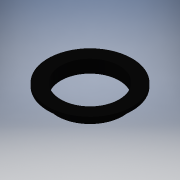
# Autodesk Inventor part: オイレスF　d25-D28-l12
Saved by Autodesk Inventor 2017.3 (Build 213256000, 256)
## iProperties
Created: 2017-03-06
Part Number: オイレスF　d25-D28-l12
Material: アセタール樹脂、黒
Document SubType Name: Modeling
Designer: 大空
Density: 1.425 g/cm^3
Appearance: 滑らか - 黒
Mass: 1.83827 g
Surface Area: 20.0748 cm^2
Volume: 1.29002 cm^3
Author: 大空
Autodesk Inventor part; units mm, degrees
ref_plane "YZ Plane" through (0, 0, 0) normal (1, 0, 0) x (0, 1, 0)
ref_plane "XZ Plane" through (0, 0, 0) normal (0, 1, 0) x (-1, 0, 0)
ref_plane "XY Plane" through (0, 0, 0) normal (0, 0, 1) x (1, 0, 0)
sketch "スケッチ1" plane through (0, 0, 0) normal (0, 0, 1) x (1, 0, 0)
  circle A0 centre (0, 0) radius 12.5
  circle A1 centre (0, 0) radius 14
  circle A2 centre (0, 0) radius 18
  dimension "d0" = 25
  dimension "d1" = 28
  dimension "d2" = 36
  constraints: 3 centre point, 3 coincident
  measures "d0" diameter of A0
  measures "d1" diameter of A1
  measures "d2" diameter of A2
extrude "押し出し1" add sketch "スケッチ1" along normal blind 1.5 contours A1 | A2
extrude "押し出し2" add sketch "スケッチ1" against normal blind 4 contours A1
